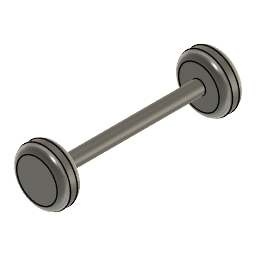
Wheels (Autodesk Fusion 360 design; units mm, degrees)
part number: 2026-03-04-16-00-43-502
Autodesk Fusion 360 part; units mm, degrees
sketch "Sketch1" plane through (0, 0, 0) normal (0, 1, 0) x (1, 0, 0)
  circle A0 centre (0, 0) radius 2.54
  dimension "d1" = 5.08
  constraint coincident A0.centre origin
  measures "d1" diameter of A0
extrude "Extrude1" add sketch "Sketch1" along normal mid plane 53.34
sketch "Sketch2" plane through (0, -26.67, 0) normal (0, -1, 0) x (1, 0, 0)
  circle A0 centre (0, 0) radius 2.54
  circle A1 centre (0, 0) radius 10.16
  dimension "d8" = 20.32
  constraint coincident A0.centre A1.centre
  measures "d8" diameter of A1
extrude "Extrude2" add sketch "Sketch2" along normal blind 7.62 contours A0 | A1
sketch "Sketch3" plane through (0, 26.67, 0) normal (0, 1, 0) x (-1, 0, 0)
  circle A0 centre (0, 0) radius 2.54
  circle A1 centre (0, 0) radius 10.16
  dimension "d9" = 20.32
  constraint coincident A0.centre A1.centre
  measures "d9" diameter of A1
extrude "Extrude3" add sketch "Sketch3" along normal blind 7.62 contours A0 | A1
fillet "Fillet1" radius 2.54 3 edges at (-9.4724, -34.29, -3.674) (9.4724, 34.29, -3.674) (-9.4724, -26.67, -3.674) 1 faces at (-10.1474, 29.21, -0.5064)
